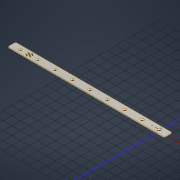
# Autodesk Inventor part: X Extrusion-Backer (350mm)
Saved by Autodesk Inventor 2022.2 (Build 262287010, 287A)
## iProperties
Created: 2022-03-23
Part Number: X Extrusion-Backer (350mm)
Material: Titan
Document SubType Name: Modeling
Designer: sleib
Density: 4.51 g/cm^3
Appearance: Titan
Author: sleib
Autodesk Inventor part; units mm, degrees
ref_plane "YZ Plane" through (0, 0, 0) normal (1, 0, 0) x (0, 1, 0)
ref_plane "XZ Plane" through (0, 0, 0) normal (0, 1, 0) x (-1, 0, 0)
ref_plane "XY Plane" through (0, 0, 0) normal (0, 0, 1) x (1, 0, 0)
sketch "ExtrusionBacker_X_350mm" plane through (0, 0, 0) normal (0, 0, 1) x (1, 0, 0)
  arc A0 (340.9999, 24.106) -> (342.9999, 26.106) centre (340.9999, 26.106) ccw
  line L0 (342.9999, 26.106) -> (342.9999, 40.106)
  arc A1 (342.9999, 40.106) -> (340.9999, 42.106) centre (340.9999, 40.106) ccw
  line L1 (340.9999, 42.106) -> (-15.0001, 42.106)
  arc A2 (-15.0001, 42.106) -> (-17.0001, 40.106) centre (-15.0001, 40.106) ccw
  line L2 (-17.0001, 40.106) -> (-17.0001, 26.106)
  arc A3 (-17.0001, 26.106) -> (-15.0001, 24.106) centre (-15.0001, 26.106) ccw
  line L3 (-15.0001, 24.106) -> (340.9999, 24.106)
  line L4 (302.2499, 37.0031) -> (307.986, 33.6914)
  line L5 (307.986, 33.6914) -> (307.986, 36.2894)
  line L6 (307.986, 36.2894) -> (302.2499, 39.6012)
  line L7 (302.2499, 39.6012) -> (302.2499, 37.0031)
  line L8 (296.5137, 37.7168) -> (296.5137, 35.1187)
  line L9 (296.5137, 35.1187) -> (307.986, 28.4952)
  line L10 (307.986, 28.4952) -> (307.986, 31.0933)
  line L11 (307.986, 31.0933) -> (296.5137, 37.7168)
  line L12 (296.5137, 32.5207) -> (296.5137, 29.9226)
  line L13 (296.5137, 29.9226) -> (302.2499, 26.6108)
  line L14 (302.2499, 26.6108) -> (302.2499, 29.2089)
  line L15 (302.2499, 29.2089) -> (296.5137, 32.5207)
  circle A4 centre (122.9999, 33.106) radius 1.7
  circle A5 centre (202.9999, 33.106) radius 1.7
  circle A6 centre (242.9999, 33.106) radius 1.7
  circle A7 centre (162.9999, 33.106) radius 1.7
  circle A8 centre (3.9999, 38.106) radius 1
  circle A9 centre (3.9999, 28.106) radius 1
  circle A10 centre (11.9999, 33.106) radius 1
  circle A11 centre (42.9999, 33.106) radius 1.7
  circle A12 centre (82.9999, 33.106) radius 1.7
  circle A13 centre (282.9999, 33.106) radius 1.7
  circle A14 centre (19.9999, 33.106) radius 1
  circle A15 centre (2.9999, 33.106) radius 1.7
  circle A16 centre (322.9999, 33.106) radius 1.7
  circle A17 centre (7.9999, 33.106) radius 1
sketch "Skizze1" plane through (0, 0, 0) normal (0, 1, 0) x (-1, 0, 0)
  arc A0 (338, -9) -> (340, -7) centre (338, -7) ccw
  line L0 (340, -7) -> (340, 7)
  arc A1 (340, 7) -> (338, 9) centre (338, 7) ccw
  line L1 (338, 9) -> (-18, 9)
  arc A2 (-18, 9) -> (-20, 7) centre (-18, 7) ccw
  line L2 (-20, 7) -> (-20, -7)
  arc A3 (-20, -7) -> (-18, -9) centre (-18, -7) ccw
  line L3 (-18, -9) -> (338, -9)
  line L4 (299.25, 3.8971) -> (304.9862, 0.5853)
  line L5 (304.9862, 0.5853) -> (304.9862, 3.1834)
  line L6 (304.9862, 3.1834) -> (299.25, 6.4952)
  line L7 (299.25, 6.4952) -> (299.25, 3.8971)
  line L8 (293.5138, 4.6108) -> (293.5138, 2.0127)
  line L9 (293.5138, 2.0127) -> (304.9862, -4.6108)
  line L10 (304.9862, -4.6108) -> (304.9862, -2.0127)
  line L11 (304.9862, -2.0127) -> (293.5138, 4.6108)
  line L12 (293.5138, -0.5853) -> (293.5138, -3.1834)
  line L13 (293.5138, -3.1834) -> (299.25, -6.4952)
  line L14 (299.25, -6.4952) -> (299.25, -3.8971)
  line L15 (299.25, -3.8971) -> (293.5138, -0.5853)
  circle A4 centre (120, 0) radius 1.7
  circle A5 centre (200, 0) radius 1.7
  circle A6 centre (240, 0) radius 1.7
  circle A7 centre (160, 0) radius 1.7
  circle A8 centre (1, 5) radius 1
  circle A9 centre (1, -5) radius 1
  circle A10 centre (9, 0) radius 1
  circle A11 centre (40, 0) radius 1.7
  circle A12 centre (80, 0) radius 1.7
  circle A13 centre (280, 0) radius 1.7
  circle A14 centre (17, 0) radius 1
  circle A15 centre (0, 0) radius 1.7
  circle A16 centre (320, 0) radius 1.7
  circle A17 centre (5, 0) radius 1
  point P0 (338, -9)
  point P1 (340, 7)
  point P2 (338, 9)
  point P3 (-18, 9)
  point P4 (-20, 7)
  point P5 (-20, -7)
  point P6 (-18, -9)
  point P7 (293.5138, -0.5853)
  point P8 (299.25, -3.8971)
  point P9 (299.25, -6.4952)
  point P10 (293.5138, -3.1834)
  point P11 (293.5138, 4.6108)
  point P12 (304.9862, -2.0127)
  point P13 (304.9862, -4.6108)
  point P14 (293.5138, 2.0127)
  point P15 (299.25, 3.8971)
  point P16 (299.25, 6.4952)
  point P17 (304.9862, 3.1834)
  point P18 (304.9862, 0.5853)
  constraints: 1 other
extrude "Extrusion1" add sketch "Skizze1" along normal blind 2
sketch "Skizze2" plane through (0, 2, 0) normal (0, 1, 0) x (1, 0, 0)
  circle A0 centre (-320, 0) radius 1.7 projected
  circle A1 centre (-280, 0) radius 1.7 projected
  circle A2 centre (-240, 0) radius 1.7 projected
  circle A3 centre (-200, 0) radius 1.7 projected
  circle A4 centre (-160, 0) radius 1.7 projected
  circle A5 centre (-120, 0) radius 1.7 projected
  circle A6 centre (-80, 0) radius 1.7 projected
  circle A7 centre (-40, 0) radius 1.7 projected
  circle A8 centre (0, 0) radius 1.7 projected
  point P0 (-81.3289, 1.9857)
  constraints: 10 coincident
hole "Bohrung1" at (-320, 2, 0) at (-280, 2, 0) at (-240, 2, 0) at (-200, 2, 0) at (-160, 2, 0) at (-120, 2, 0) at (-80, 2, 0) at (-40, 2, 0) at (0, 2, 0) direction (0, -1, 0) diameter 3.4 end through all countersink diameter 7.5 countersink angle 90 clearance for "Innensechskant-Senkkopfschraube DIN EN ISO 10642" size "M3" standard "DIN"
